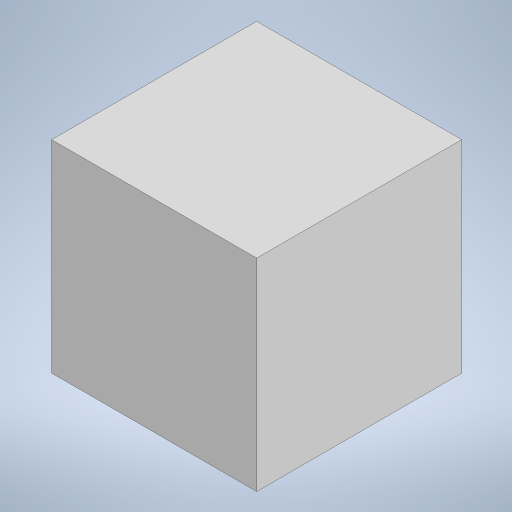
# Autodesk Inventor part: Part1 ZAID
Saved by Autodesk Inventor 2023 (Build 270158030, 158C)
## iProperties
Created: 2023-04-28
Part Number: Part1 ZAID
Material: Generic
Document SubType Name: Modeling
Designer: 22165
Density: 1 g/cm^3
Appearance: Default
Author: 22165
Autodesk Inventor part; units mm, degrees
ref_plane "YZ Plane" through (0, 0, 0) normal (1, 0, 0) x (0, 1, 0)
ref_plane "XZ Plane" through (0, 0, 0) normal (0, 1, 0) x (-1, 0, 0)
ref_plane "XY Plane" through (0, 0, 0) normal (0, 0, 1) x (1, 0, 0)
sketch "Sketch1" plane through (0, 0, 0) normal (0, 0, 1) x (1, 0, 0)
  line L0 (0, 0) -> (140, 0)
  line L1 (140, 0) -> (140, -140)
  line L2 (140, -140) -> (0, -140)
  line L3 (0, -140) -> (0, 0)
  dimension "d0" = 140
  dimension "d1" = 140
  constraints: 8 end point, 2 parallel, 1 horizontal, 1 perpendicular
  measures "d0" distance of L1.end L2.end
  measures "d1" distance of L0.end L1.end
extrude "Extrusion1" add sketch "Sketch1" along normal blind 140
shell "Shell1" thickness 2 outward yes removed faces 1 at (46.6667, -140, 46.6667)
sketch "Sketch2" plane through (0, 0, -2) normal (0, 0, -1) x (-1, 0, 0)
  line L0 (-39, -10) -> (-101, -10)
  line L1 (-101, -10) -> (-101, -128)
  line L2 (-101, -128) -> (-39, -128)
  line L3 (-39, -128) -> (-39, -10)
  line L4 (-140, 0) -> (0, 0) projected
  line L5 (-140, -140) -> (-140, 0) projected
  point P0 (-101, -69)
  dimension "d5" = 118
  dimension "d6" = 62
  dimension "d7" = 10
  dimension "d8" = 39
  constraints: 8 end point, 2 parallel, 1 horizontal, 1 midpoint, 1 perpendicular
  measures "d5" distance of L2.end L0.start
  measures "d6" distance of L0.start L0.end
  measures "d7" distance between parallel lines of L0 L4
  measures "d8" distance from line of L5 point (-101, -69)
extrude "Extrusion2" cut sketch "Sketch2" against normal blind 20
sketch "Sketch3" plane through (-2, -140, -2) normal (-1, 0, 0) x (0, 0, 1)
  line L0 (3.4931, 8.4292) -> (19.1435, 8.4292) construction
  line L1 (19.1435, 8.4292) -> (19.1435, 1.9288) construction
  line L2 (19.1435, 1.9288) -> (3.4931, 1.9288) construction
  line L3 (3.4931, 1.9288) -> (3.4931, 8.4292) construction
  spline S0 degree 2 poles (7.6615, 6.3923) (7.3247, 6.3923) (7.1615, 6.7502) knots 0 0 0 1 1 1
  spline S1 degree 2 poles (7.1615, 6.7502) (7.0878, 6.9239) (7.0089, 6.9555) knots 0 0 0 1 1 1
  spline S2 degree 2 poles (7.0089, 6.9555) (6.951, 6.9818) (6.7089, 6.9818) knots 0 0 0 1 1 1
  spline S3 degree 2 poles (6.7089, 6.9818) (6.2352, 6.9818) (5.6141, 6.2397) knots 0 0 0 1 1 1
  spline S4 degree 2 poles (5.6141, 6.2397) (4.7404, 5.2081) (4.7404, 4.3029) knots 0 0 0 1 1 1
  spline S5 degree 2 poles (4.7404, 4.3029) (4.7404, 3.8923) (5.2931, 3.3029) (5.6773, 3.3029) knots 0 0 0 1 2 2 2
  spline S6 degree 2 poles (5.6773, 3.3029) (6.051, 3.3029) (6.4352, 3.4976) knots 0 0 0 1 1 1
  spline S7 degree 2 poles (6.4352, 3.4976) (6.572, 3.5713) (7.0089, 3.8713) knots 0 0 0 1 1 1
  spline S8 degree 2 poles (7.0089, 3.8713) (7.3036, 4.066) (7.4562, 4.066) knots 0 0 0 1 1 1
  spline S9 degree 2 poles (7.4562, 4.066) (7.6826, 4.066) (7.8404, 3.8976) knots 0 0 0 1 1 1
  spline S10 degree 2 poles (7.8404, 3.8976) (7.9878, 3.745) (7.9878, 3.545) knots 0 0 0 1 1 1
  spline S11 degree 2 poles (7.9878, 3.545) (7.9878, 3.3239) (7.7931, 3.1555) knots 0 0 0 1 1 1
  spline S12 degree 2 poles (7.7931, 3.1555) (6.751, 2.2818) (5.6773, 2.2818) knots 0 0 0 1 1 1
  spline S13 degree 2 poles (5.6773, 2.2818) (4.8247, 2.2818) (4.2404, 2.9029) knots 0 0 0 1 1 1
  spline S14 degree 2 poles (4.2404, 2.9029) (3.6826, 3.4976) (3.6826, 4.3029) knots 0 0 0 1 1 1
  spline S15 degree 2 poles (3.6826, 4.3029) (3.6826, 5.5713) (4.7878, 6.8871) knots 0 0 0 1 1 1
  spline S16 degree 2 poles (4.7878, 6.8871) (5.7299, 8.0029) (6.7089, 8.0029) knots 0 0 0 1 1 1
  spline S17 degree 2 poles (6.7089, 8.0029) (6.8773, 8.0029) (7.1457, 7.9818) (7.2457, 7.9555) knots 0 0 0 1 2 2 2
  spline S18 degree 2 poles (7.2457, 7.9555) (7.4141, 8.1186) (7.6457, 8.1186) knots 0 0 0 1 1 1
  spline S19 degree 2 poles (7.6457, 8.1186) (8.0352, 8.1186) (8.1247, 7.6765) knots 0 0 0 1 1 1
  spline S20 degree 2 poles (8.1247, 7.6765) (8.1878, 7.3607) (8.1878, 6.9397) knots 0 0 0 1 1 1
  spline S21 degree 2 poles (8.1878, 6.9397) (8.1878, 6.7502) (8.0773, 6.5976) knots 0 0 0 1 1 1
  spline S22 degree 2 poles (8.0773, 6.5976) (7.9352, 6.3923) (7.6615, 6.3923) knots 0 0 0 1 1 1
  spline S23 degree 2 poles (10.2194, 2.1502) (9.5194, 2.1502) (9.0194, 2.6292) knots 0 0 0 1 1 1
  spline S24 degree 2 poles (9.0194, 2.6292) (8.4668, 3.1555) (8.4404, 4.0292) knots 0 0 0 1 1 1
  spline S25 degree 2 poles (8.4404, 4.0292) (8.4141, 4.866) (8.8983, 5.5186) knots 0 0 0 1 1 1
  spline S26 degree 2 poles (8.8983, 5.5186) (9.472, 6.2871) (10.4983, 6.2871) knots 0 0 0 1 1 1
  spline S27 degree 2 poles (10.4983, 6.2871) (11.251, 6.2871) (11.6983, 5.6818) knots 0 0 0 1 1 1
  spline S28 degree 2 poles (11.6983, 5.6818) (12.0983, 5.1397) (12.0983, 4.3344) knots 0 0 0 1 1 1
  spline S29 degree 2 poles (12.0983, 4.3344) (12.0983, 3.4607) (11.6299, 2.8397) knots 0 0 0 1 1 1
  spline S30 degree 2 poles (11.6299, 2.8397) (11.1036, 2.1502) (10.2194, 2.1502) knots 0 0 0 1 1 1
  spline S31 degree 2 poles (10.451, 5.2923) (9.9826, 5.2976) (9.7141, 4.8713) knots 0 0 0 1 1 1
  spline S32 degree 2 poles (9.7141, 4.8713) (9.4878, 4.5134) (9.4878, 4.0344) knots 0 0 0 1 1 1
  spline S33 degree 2 poles (9.4878, 4.0344) (9.4878, 3.5765) (9.7457, 3.3397) knots 0 0 0 1 1 1
  spline S34 degree 2 poles (9.7457, 3.3397) (9.951, 3.145) (10.2194, 3.145) knots 0 0 0 1 1 1
  spline S35 degree 2 poles (10.2194, 3.145) (10.551, 3.145) (10.7931, 3.366) knots 0 0 0 1 1 1
  spline S36 degree 2 poles (10.7931, 3.366) (11.0668, 3.6292) (11.0878, 4.0713) knots 0 0 0 1 1 1
  spline S37 degree 2 poles (11.0878, 4.0713) (11.1352, 5.2871) (10.451, 5.2923) knots 0 0 0 1 1 1
  spline S38 degree 2 poles (13.9141, 4.1397) (13.9141, 3.9239) (13.9404, 2.9713) (13.9404, 2.7607) knots 0 0 0 1 2 2 2
  spline S39 degree 2 poles (13.9404, 2.7607) (13.9404, 2.5397) (13.6457, 2.2555) (13.4194, 2.2555) knots 0 0 0 1 2 2 2
  spline S40 degree 2 poles (13.4194, 2.2555) (13.1931, 2.2555) (12.8983, 2.5397) (12.8983, 2.7607) knots 0 0 0 1 2 2 2
  spline S41 degree 2 poles (12.8983, 2.7607) (12.8983, 2.9713) (12.872, 3.9239) (12.872, 4.1397) knots 0 0 0 1 2 2 2
  spline S42 degree 2 poles (12.872, 4.1397) (12.872, 4.4765) (12.9457, 5.4923) (12.9457, 5.8292) knots 0 0 0 1 2 2 2
  spline S43 degree 2 poles (12.9457, 5.8292) (12.9457, 6.045) (13.2404, 6.3292) (13.4668, 6.3292) knots 0 0 0 1 2 2 2
  spline S44 degree 2 poles (13.4668, 6.3292) (13.6931, 6.3292) (13.9878, 6.045) (13.9878, 5.8292) knots 0 0 0 1 2 2 2
  spline S45 degree 2 poles (13.9878, 5.8292) (13.9878, 5.4923) (13.9141, 4.4765) (13.9141, 4.1397) knots 0 0 0 1 2 2 2
  spline S46 degree 2 poles (13.5931, 6.9081) (13.351, 6.9081) (12.9983, 7.2344) (12.9983, 7.466) knots 0 0 0 1 2 2 2
  spline S47 degree 2 poles (12.9983, 7.466) (12.9983, 7.6976) (13.351, 8.0239) (13.5931, 8.0239) knots 0 0 0 1 2 2 2
  spline S48 degree 2 poles (13.5931, 8.0239) (13.8352, 8.0239) (14.1878, 7.6976) (14.1878, 7.466) knots 0 0 0 1 2 2 2
  spline S49 degree 2 poles (14.1878, 7.466) (14.1878, 7.2344) (13.8352, 6.9081) (13.5931, 6.9081) knots 0 0 0 1 2 2 2
  spline S50 degree 2 poles (17.872, 2.1029) (17.4036, 2.1029) (17.351, 2.5607) knots 0 0 0 1 1 1
  spline S51 degree 2 poles (17.351, 2.5607) (17.3036, 2.9502) (17.251, 3.3397) knots 0 0 0 1 1 1
  spline S52 degree 2 poles (17.251, 3.3397) (17.1983, 3.7555) (17.1983, 4.1239) knots 0 0 0 1 1 1
  spline S53 degree 2 poles (17.1983, 4.1239) (17.1983, 4.2239) (17.2194, 4.6976) (17.2194, 4.7976) knots 0 0 0 1 2 2 2
  spline S54 degree 2 poles (17.2194, 4.7976) (17.2194, 4.8239) (17.2352, 5.0397) (17.2352, 5.1029) knots 0 0 0 1 2 2 2
  spline S55 degree 2 poles (17.2352, 5.1029) (17.2352, 5.4186) (17.0826, 5.4186) knots 0 0 0 1 1 1
  spline S56 degree 2 poles (17.0826, 5.4186) (16.7615, 5.4186) (16.1404, 4.5871) (15.9668, 3.9502) knots 0 0 0 1 2 2 2
  spline S57 degree 2 poles (15.9668, 3.9502) (15.9615, 3.8186) (15.9352, 3.6081) knots 0 0 0 1 1 1
  spline S58 degree 2 poles (15.9352, 3.6081) (15.9141, 3.4344) (15.9141, 3.266) knots 0 0 0 1 1 1
  spline S59 degree 2 poles (15.9141, 3.266) (15.9141, 3.1607) (15.8668, 2.7239) (15.8668, 2.6134) knots 0 0 0 1 2 2 2
  spline S60 degree 2 poles (15.8668, 2.6134) (15.8668, 2.3923) (15.5668, 2.1029) (15.3404, 2.1029) knots 0 0 0 1 2 2 2
  spline S61 degree 2 poles (15.3404, 2.1029) (15.1141, 2.1029) (14.8194, 2.3923) (14.8194, 2.6081) knots 0 0 0 1 2 2 2
  spline S62 degree 2 poles (14.8194, 2.6081) (14.8194, 2.7186) (14.772, 3.1502) (14.772, 3.2607) knots 0 0 0 1 2 2 2
  spline S63 degree 2 poles (14.772, 3.2607) (14.772, 3.6292) (14.8773, 4.945) (14.8773, 5.3134) knots 0 0 0 1 2 2 2
  spline S64 degree 2 poles (14.8773, 5.3134) (14.8773, 5.4292) (14.851, 5.8871) (14.851, 5.9976) knots 0 0 0 1 2 2 2
  spline S65 degree 2 poles (14.851, 5.9976) (14.851, 6.2134) (15.1562, 6.4923) (15.3826, 6.4923) knots 0 0 0 1 2 2 2
  spline S66 degree 2 poles (15.3826, 6.4923) (15.8773, 6.4923) (15.9089, 5.8976) knots 0 0 0 1 1 1
  line L4 (15.9089, 5.8976) -> (15.9141, 5.8607)
  spline S67 degree 2 poles (15.9141, 5.8607) (16.4668, 6.4134) (17.0773, 6.4134) knots 0 0 0 1 1 1
  spline S68 degree 2 poles (17.0773, 6.4134) (17.7878, 6.4134) (18.0615, 5.8186) knots 0 0 0 1 1 1
  spline S69 degree 2 poles (18.0615, 5.8186) (18.2404, 5.4186) (18.2404, 4.6186) knots 0 0 0 1 1 1
  line L5 (18.2404, 4.6186) -> (18.2404, 4.3502)
  spline S70 degree 2 poles (18.2404, 4.3502) (18.2352, 4.1765) (18.2352, 4.1081) knots 0 0 0 1 1 1
  spline S71 degree 2 poles (18.2352, 4.1081) (18.2352, 3.8134) (18.3983, 2.8818) (18.3983, 2.5923) knots 0 0 0 1 2 2 2
  spline S72 degree 2 poles (18.3983, 2.5923) (18.3983, 2.3818) (18.0931, 2.1029) (17.872, 2.1029) knots 0 0 0 1 2 2 2
  spline S73 degree 2 poles (20.6826, 2.1344) (19.851, 2.1344) (19.2931, 2.6081) knots 0 0 0 1 1 1
  spline S74 degree 2 poles (19.2931, 2.6081) (18.6983, 3.1029) (18.6983, 3.9186) knots 0 0 0 1 1 1
  spline S75 degree 2 poles (18.6983, 3.9186) (18.6983, 4.6713) (19.2299, 5.4713) knots 0 0 0 1 1 1
  spline S76 degree 2 poles (19.2299, 5.4713) (19.8352, 6.3818) (20.6352, 6.3818) knots 0 0 0 1 1 1
  spline S77 degree 2 poles (20.6352, 6.3818) (21.0247, 6.3818) (21.551, 6.1713) knots 0 0 0 1 1 1
  spline S78 degree 2 poles (21.551, 6.1713) (22.1878, 5.9081) (22.1878, 5.5713) knots 0 0 0 1 1 1
  spline S79 degree 2 poles (22.1878, 5.5713) (22.1878, 5.3871) (22.0615, 5.2397) knots 0 0 0 1 1 1
  spline S80 degree 2 poles (22.0615, 5.2397) (21.9247, 5.0871) (21.7089, 5.0871) knots 0 0 0 1 1 1
  spline S81 degree 2 poles (21.7089, 5.0871) (21.5457, 5.0871) (21.0878, 5.4397) (20.6299, 5.4397) knots 0 0 0 1 2 2 2
  spline S82 degree 2 poles (20.6299, 5.4397) (20.3404, 5.4397) (20.0036, 4.8713) knots 0 0 0 1 1 1
  spline S83 degree 2 poles (20.0036, 4.8713) (19.6773, 4.3186) (19.6773, 3.9186) knots 0 0 0 1 1 1
  spline S84 degree 2 poles (19.6773, 3.9186) (19.6773, 3.5239) (19.9668, 3.2976) knots 0 0 0 1 1 1
  spline S85 degree 2 poles (19.9668, 3.2976) (20.2352, 3.0818) (20.6826, 3.0818) knots 0 0 0 1 1 1
  spline S86 degree 2 poles (20.6826, 3.0818) (20.9352, 3.0818) (21.6668, 3.466) (21.7668, 3.466) knots 0 0 0 1 2 2 2
  spline S87 degree 2 poles (21.7668, 3.466) (21.972, 3.466) (22.2615, 3.1713) (22.2615, 2.9818) knots 0 0 0 1 2 2 2
  spline S88 degree 2 poles (22.2615, 2.9818) (22.2615, 2.6871) (21.6194, 2.3923) knots 0 0 0 1 1 1
  spline S89 degree 2 poles (21.6194, 2.3923) (21.0457, 2.1344) (20.6826, 2.1344) knots 0 0 0 1 1 1
  spline S90 degree 2 poles (24.4773, 2.1502) (23.7773, 2.1502) (23.2773, 2.6292) knots 0 0 0 1 1 1
  spline S91 degree 2 poles (23.2773, 2.6292) (22.7247, 3.1555) (22.6983, 4.0292) knots 0 0 0 1 1 1
  spline S92 degree 2 poles (22.6983, 4.0292) (22.672, 4.866) (23.1562, 5.5186) knots 0 0 0 1 1 1
  spline S93 degree 2 poles (23.1562, 5.5186) (23.7299, 6.2871) (24.7562, 6.2871) knots 0 0 0 1 1 1
  spline S94 degree 2 poles (24.7562, 6.2871) (25.5089, 6.2871) (25.9562, 5.6818) knots 0 0 0 1 1 1
  spline S95 degree 2 poles (25.9562, 5.6818) (26.3562, 5.1397) (26.3562, 4.3344) knots 0 0 0 1 1 1
  spline S96 degree 2 poles (26.3562, 4.3344) (26.3562, 3.4607) (25.8878, 2.8397) knots 0 0 0 1 1 1
  spline S97 degree 2 poles (25.8878, 2.8397) (25.3615, 2.1502) (24.4773, 2.1502) knots 0 0 0 1 1 1
  spline S98 degree 2 poles (24.7089, 5.2923) (24.2404, 5.2976) (23.972, 4.8713) knots 0 0 0 1 1 1
  spline S99 degree 2 poles (23.972, 4.8713) (23.7457, 4.5134) (23.7457, 4.0344) knots 0 0 0 1 1 1
  spline S100 degree 2 poles (23.7457, 4.0344) (23.7457, 3.5765) (24.0036, 3.3397) knots 0 0 0 1 1 1
  spline S101 degree 2 poles (24.0036, 3.3397) (24.2089, 3.145) (24.4773, 3.145) knots 0 0 0 1 1 1
  spline S102 degree 2 poles (24.4773, 3.145) (24.8089, 3.145) (25.051, 3.366) knots 0 0 0 1 1 1
  spline S103 degree 2 poles (25.051, 3.366) (25.3247, 3.6292) (25.3457, 4.0713) knots 0 0 0 1 1 1
  spline S104 degree 2 poles (25.3457, 4.0713) (25.3931, 5.2871) (24.7089, 5.2923) knots 0 0 0 1 1 1
  spline S105 degree 2 poles (28.151, 2.9239) (28.151, 2.2081) (27.6299, 2.2081) knots 0 0 0 1 1 1
  spline S106 degree 2 poles (27.6299, 2.2081) (27.4036, 2.2081) (27.1089, 2.4976) (27.1089, 2.7239) knots 0 0 0 1 2 2 2
  line L6 (27.1089, 2.7239) -> (27.1089, 7.9397)
  spline S107 degree 2 poles (27.1089, 7.9397) (27.1089, 8.1607) (27.2668, 8.3029) knots 0 0 0 1 1 1
  spline S108 degree 2 poles (27.2668, 8.3029) (27.4194, 8.4292) (27.6404, 8.4292) knots 0 0 0 1 1 1
  spline S109 degree 2 poles (27.6404, 8.4292) (27.8615, 8.4292) (28.151, 8.1607) (28.151, 7.9397) knots 0 0 0 1 2 2 2
  line L7 (28.151, 7.9397) -> (28.151, 2.9239)
  spline S110 degree 2 poles (30.2668, 2.9239) (30.2668, 2.2081) (29.7457, 2.2081) knots 0 0 0 1 1 1
  spline S111 degree 2 poles (29.7457, 2.2081) (29.5194, 2.2081) (29.2247, 2.4976) (29.2247, 2.7239) knots 0 0 0 1 2 2 2
  line L8 (29.2247, 2.7239) -> (29.2247, 7.9397)
  spline S112 degree 2 poles (29.2247, 7.9397) (29.2247, 8.1607) (29.3826, 8.3029) knots 0 0 0 1 1 1
  spline S113 degree 2 poles (29.3826, 8.3029) (29.5352, 8.4292) (29.7562, 8.4292) knots 0 0 0 1 1 1
  spline S114 degree 2 poles (29.7562, 8.4292) (29.9773, 8.4292) (30.2668, 8.1607) (30.2668, 7.9397) knots 0 0 0 1 2 2 2
  line L9 (30.2668, 7.9397) -> (30.2668, 2.9239)
  spline S115 degree 2 poles (33.1247, 2.1976) (32.2194, 2.1976) (31.6457, 2.6292) knots 0 0 0 1 1 1
  spline S116 degree 2 poles (31.6457, 2.6292) (31.0141, 3.1029) (31.0141, 3.9713) knots 0 0 0 1 1 1
  spline S117 degree 2 poles (31.0141, 3.9713) (31.0141, 4.9239) (31.5141, 5.5871) knots 0 0 0 1 1 1
  spline S118 degree 2 poles (31.5141, 5.5871) (32.0773, 6.3186) (33.0194, 6.3186) knots 0 0 0 1 1 1
  spline S119 degree 2 poles (33.0194, 6.3186) (33.6773, 6.3186) (34.1141, 6.1081) knots 0 0 0 1 1 1
  spline S120 degree 2 poles (34.1141, 6.1081) (34.6826, 5.8292) (34.6826, 5.2397) knots 0 0 0 1 1 1
  spline S121 degree 2 poles (34.6826, 5.2397) (34.6826, 4.8239) (34.2194, 4.5029) knots 0 0 0 1 1 1
  spline S122 degree 2 poles (34.2194, 4.5029) (34.0089, 4.3555) (33.372, 4.0713) knots 0 0 0 1 1 1
  line L10 (33.372, 4.0713) -> (32.0983, 3.5081)
  spline S123 degree 2 poles (32.0983, 3.5081) (32.2773, 3.3134) (32.7931, 3.1134) (33.1247, 3.1134) knots 0 0 0 1 2 2 2
  spline S124 degree 2 poles (33.1247, 3.1134) (33.6299, 3.1134) (33.9773, 3.3239) knots 0 0 0 1 1 1
  spline S125 degree 2 poles (33.9773, 3.3239) (34.2931, 3.5081) (34.4826, 3.5081) knots 0 0 0 1 1 1
  spline S126 degree 2 poles (34.4826, 3.5081) (34.872, 3.5081) (34.872, 3.1292) knots 0 0 0 1 1 1
  spline S127 degree 2 poles (34.872, 3.1292) (34.872, 2.6976) (34.2404, 2.4239) knots 0 0 0 1 1 1
  spline S128 degree 2 poles (34.2404, 2.4239) (33.7141, 2.1976) (33.1247, 2.1976) knots 0 0 0 1 1 1
  spline S129 degree 2 poles (33.0247, 5.4029) (32.672, 5.4029) (32.1773, 4.9344) (32.0247, 4.466) knots 0 0 0 1 2 2 2
  spline S130 degree 2 poles (32.0247, 4.466) (32.451, 4.6502) (32.872, 4.8344) knots 0 0 0 1 1 1
  spline S131 degree 2 poles (32.872, 4.8344) (33.3826, 5.0607) (33.6826, 5.2607) knots 0 0 0 1 1 1
  spline S132 degree 2 poles (33.6826, 5.2607) (33.4299, 5.4029) (33.0247, 5.4029) knots 0 0 0 1 1 1
  spline S133 degree 2 poles (37.2773, 2.1344) (36.4457, 2.1344) (35.8878, 2.6081) knots 0 0 0 1 1 1
  spline S134 degree 2 poles (35.8878, 2.6081) (35.2931, 3.1029) (35.2931, 3.9186) knots 0 0 0 1 1 1
  spline S135 degree 2 poles (35.2931, 3.9186) (35.2931, 4.6713) (35.8247, 5.4713) knots 0 0 0 1 1 1
  spline S136 degree 2 poles (35.8247, 5.4713) (36.4299, 6.3818) (37.2299, 6.3818) knots 0 0 0 1 1 1
  spline S137 degree 2 poles (37.2299, 6.3818) (37.6194, 6.3818) (38.1457, 6.1713) knots 0 0 0 1 1 1
  spline S138 degree 2 poles (38.1457, 6.1713) (38.7826, 5.9081) (38.7826, 5.5713) knots 0 0 0 1 1 1
  spline S139 degree 2 poles (38.7826, 5.5713) (38.7826, 5.3871) (38.6562, 5.2397) knots 0 0 0 1 1 1
  spline S140 degree 2 poles (38.6562, 5.2397) (38.5194, 5.0871) (38.3036, 5.0871) knots 0 0 0 1 1 1
  spline S141 degree 2 poles (38.3036, 5.0871) (38.1404, 5.0871) (37.6826, 5.4397) (37.2247, 5.4397) knots 0 0 0 1 2 2 2
  spline S142 degree 2 poles (37.2247, 5.4397) (36.9352, 5.4397) (36.5983, 4.8713) knots 0 0 0 1 1 1
  spline S143 degree 2 poles (36.5983, 4.8713) (36.272, 4.3186) (36.272, 3.9186) knots 0 0 0 1 1 1
  spline S144 degree 2 poles (36.272, 3.9186) (36.272, 3.5239) (36.5615, 3.2976) knots 0 0 0 1 1 1
  spline S145 degree 2 poles (36.5615, 3.2976) (36.8299, 3.0818) (37.2773, 3.0818) knots 0 0 0 1 1 1
  spline S146 degree 2 poles (37.2773, 3.0818) (37.5299, 3.0818) (38.2615, 3.466) (38.3615, 3.466) knots 0 0 0 1 2 2 2
  spline S147 degree 2 poles (38.3615, 3.466) (38.5668, 3.466) (38.8562, 3.1713) (38.8562, 2.9818) knots 0 0 0 1 2 2 2
  spline S148 degree 2 poles (38.8562, 2.9818) (38.8562, 2.6871) (38.2141, 2.3923) knots 0 0 0 1 1 1
  spline S149 degree 2 poles (38.2141, 2.3923) (37.6404, 2.1344) (37.2773, 2.1344) knots 0 0 0 1 1 1
  spline S150 degree 2 poles (42.1773, 5.4134) (42.0983, 5.4134) (41.8826, 5.4239) (41.8036, 5.4239) knots 0 0 0 1 2 2 2
  spline S151 degree 2 poles (41.8036, 5.4239) (41.651, 5.4239) (41.4457, 5.3923) knots 0 0 0 1 1 1
  spline S152 degree 2 poles (41.4457, 5.3923) (41.5141, 3.866) (41.5141, 3.3976) knots 0 0 0 1 1 1
  spline S153 degree 2 poles (41.5141, 3.3976) (41.5141, 3.3502) (41.5194, 3.0818) (41.5194, 2.9976) knots 0 0 0 1 2 2 2
  spline S154 degree 2 poles (41.5194, 2.9976) (41.5194, 2.1292) (40.972, 2.1292) knots 0 0 0 1 1 1
  spline S155 degree 2 poles (40.972, 2.1292) (40.7615, 2.1292) (40.6141, 2.2555) knots 0 0 0 1 1 1
  spline S156 degree 2 poles (40.6141, 2.2555) (40.4457, 2.3923) (40.4457, 2.5976) knots 0 0 0 1 1 1
  spline S157 degree 2 poles (40.4457, 2.5976) (40.4457, 2.7344) (40.4668, 3.2765) (40.4668, 3.4134) knots 0 0 0 1 2 2 2
  spline S158 degree 2 poles (40.4668, 3.4134) (40.4668, 3.8713) (40.4036, 5.3713) knots 0 0 0 1 1 1
  spline S159 degree 2 poles (40.4036, 5.3713) (40.1668, 5.3818) (39.2194, 5.4871) (39.2194, 5.9239) knots 0 0 0 1 2 2 2
  spline S160 degree 2 poles (39.2194, 5.9239) (39.2194, 6.1344) (39.5089, 6.4292) (39.7352, 6.4292) knots 0 0 0 1 2 2 2
  spline S161 degree 2 poles (39.7352, 6.4292) (39.872, 6.4292) (40.3773, 6.3818) knots 0 0 0 1 1 1
  spline S162 degree 2 poles (40.3773, 6.3818) (40.372, 6.5029) (40.3615, 6.7818) knots 0 0 0 1 1 1
  spline S163 degree 2 poles (40.3615, 6.7818) (40.3457, 7.0239) (40.3457, 7.1555) knots 0 0 0 1 1 1
  spline S164 degree 2 poles (40.3457, 7.1555) (40.3457, 7.366) (40.6562, 7.645) (40.872, 7.645) knots 0 0 0 1 2 2 2
  spline S165 degree 2 poles (40.872, 7.645) (41.4299, 7.645) (41.4299, 6.7081) knots 0 0 0 1 1 1
  line L11 (41.4299, 6.7081) -> (41.4247, 6.3976)
  spline S166 degree 2 poles (41.4247, 6.3976) (41.6562, 6.4292) (41.8036, 6.4292) knots 0 0 0 1 1 1
  spline S167 degree 2 poles (41.8036, 6.4292) (42.2404, 6.4292) (42.3983, 6.3713) knots 0 0 0 1 1 1
  spline S168 degree 2 poles (42.3983, 6.3713) (42.6983, 6.266) (42.6983, 5.9134) knots 0 0 0 1 1 1
  spline S169 degree 2 poles (42.6983, 5.9134) (42.6983, 5.6976) (42.4036, 5.4134) (42.1773, 5.4134) knots 0 0 0 1 2 2 2
  spline S170 degree 2 poles (44.7141, 2.1502) (44.0141, 2.1502) (43.5141, 2.6292) knots 0 0 0 1 1 1
  spline S171 degree 2 poles (43.5141, 2.6292) (42.9615, 3.1555) (42.9352, 4.0292) knots 0 0 0 1 1 1
  spline S172 degree 2 poles (42.9352, 4.0292) (42.9089, 4.866) (43.3931, 5.5186) knots 0 0 0 1 1 1
  spline S173 degree 2 poles (43.3931, 5.5186) (43.9668, 6.2871) (44.9931, 6.2871) knots 0 0 0 1 1 1
  spline S174 degree 2 poles (44.9931, 6.2871) (45.7457, 6.2871) (46.1931, 5.6818) knots 0 0 0 1 1 1
  spline S175 degree 2 poles (46.1931, 5.6818) (46.5931, 5.1397) (46.5931, 4.3344) knots 0 0 0 1 1 1
  spline S176 degree 2 poles (46.5931, 4.3344) (46.5931, 3.4607) (46.1247, 2.8397) knots 0 0 0 1 1 1
  spline S177 degree 2 poles (46.1247, 2.8397) (45.5983, 2.1502) (44.7141, 2.1502) knots 0 0 0 1 1 1
  spline S178 degree 2 poles (44.9457, 5.2923) (44.4773, 5.2976) (44.2089, 4.8713) knots 0 0 0 1 1 1
  spline S179 degree 2 poles (44.2089, 4.8713) (43.9826, 4.5134) (43.9826, 4.0344) knots 0 0 0 1 1 1
  spline S180 degree 2 poles (43.9826, 4.0344) (43.9826, 3.5765) (44.2404, 3.3397) knots 0 0 0 1 1 1
  spline S181 degree 2 poles (44.2404, 3.3397) (44.4457, 3.145) (44.7141, 3.145) knots 0 0 0 1 1 1
  spline S182 degree 2 poles (44.7141, 3.145) (45.0457, 3.145) (45.2878, 3.366) knots 0 0 0 1 1 1
  spline S183 degree 2 poles (45.2878, 3.366) (45.5615, 3.6292) (45.5826, 4.0713) knots 0 0 0 1 1 1
  spline S184 degree 2 poles (45.5826, 4.0713) (45.6299, 5.2871) (44.9457, 5.2923) knots 0 0 0 1 1 1
  spline S185 degree 2 poles (50.3878, 5.0923) (50.3562, 4.5134) (49.8668, 4.5134) knots 0 0 0 1 1 1
  spline S186 degree 2 poles (49.8668, 4.5134) (49.3931, 4.5134) (49.3931, 5.0029) knots 0 0 0 1 1 1
  line L12 (49.3931, 5.0029) -> (49.372, 5.3871)
  spline S187 degree 2 poles (49.372, 5.3871) (48.5247, 5.2502) (48.1562, 4.5134) knots 0 0 0 1 1 1
  line L13 (48.1562, 4.5134) -> (48.1615, 2.6186)
  spline S188 degree 2 poles (48.1615, 2.6186) (48.1615, 2.4029) (47.8668, 2.1186) (47.6404, 2.1186) knots 0 0 0 1 2 2 2
  spline S189 degree 2 poles (47.6404, 2.1186) (47.4036, 2.1186) (47.2773, 2.2713) knots 0 0 0 1 1 1
  spline S190 degree 2 poles (47.2773, 2.2713) (47.1562, 2.4081) (47.1562, 2.6186) knots 0 0 0 1 1 1
  line L14 (47.1562, 2.6186) -> (47.1562, 5.0871)
  spline S191 degree 2 poles (47.1562, 5.0871) (47.1562, 5.2081) (47.172, 5.6713) (47.172, 5.7871) knots 0 0 0 1 2 2 2
  spline S192 degree 2 poles (47.172, 5.7871) (47.172, 5.9976) (47.4247, 6.2818) (47.6562, 6.2818) knots 0 0 0 1 2 2 2
  spline S193 degree 2 poles (47.6562, 6.2818) (48.0773, 6.2818) (48.1562, 5.8502) knots 0 0 0 1 1 1
  spline S194 degree 2 poles (48.1562, 5.8502) (48.8247, 6.3502) (49.6404, 6.3502) knots 0 0 0 1 1 1
  spline S195 degree 2 poles (49.6404, 6.3502) (50.3931, 6.3502) (50.3931, 5.345) knots 0 0 0 1 1 1
  spline S196 degree 2 poles (50.3931, 5.345) (50.3931, 5.1502) (50.3878, 5.0923) knots 0 0 0 1 1 1
  point P0 (2, 140)
  constraints: 2 other
extrude "Extrusion3" add sketch "Sketch3" along normal blind 1
body "Solid1"
